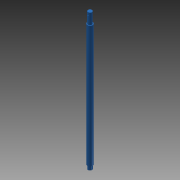
# Autodesk Inventor part: 砂轮轴
Saved by Autodesk Inventor 2015 (Build 190159000, 159)
## iProperties
Created: 2017-05-16
Part Number: 砂轮轴
Material: 常规
Document SubType Name: Modeling
Designer: Administrator
Density: 1 g/cm^3
Appearance: 青色
Author: Administrator
Autodesk Inventor part; units mm, degrees
ref_plane "YZ Plane" through (0, 0, 0) normal (1, 0, 0) x (0, 1, 0)
sketch "草图1" plane through (0, 0, 0) normal (0, 0, 1) x (1, 0, 0)
  circle A0 centre (0, 0) radius 10
  dimension "d0" = 20
  constraints: 1 centre point, 1 coincident
  measures "d0" diameter of A0
extrude "拉伸1" add sketch "草图1" along normal blind 450
sketch "草图2" plane through (0, 0, 450) normal (0, 0, 1) x (1, 0, 0)
  circle A0 centre (0, 0) radius 7.5
  dimension "d3" = 15
  constraints: 1 centre point, 1 coincident
  measures "d3" diameter of A0
extrude "拉伸2" add sketch "草图2" along normal blind 40
sketch "草图3" plane through (0, 0, 0) normal (0, 0, -1) x (-1, 0, 0)
  circle A0 centre (0, 0) radius 7.5
  dimension "d6" = 15
  constraints: 1 centre point, 1 coincident
  measures "d6" diameter of A0
extrude "拉伸3" add sketch "草图3" along normal blind 15
chamfer "倒角1" distance 0.5 angle 45 1 edges at (7.5, 0, -15)
ref_plane "工作平面1" through (0, 10, 0) normal (0, 1, 0) x (-1, 0, 0)
sketch "草图4" plane through (0, 10, 0) normal (0, 1, 0) x (-1, 0, 0)
  line L0 (3, 392) -> (-3, 392)
  line L1 (-3, 392) -> (-3, 408)
  line L2 (-3, 408) -> (3, 408)
  line L3 (3, 408) -> (3, 392)
  arc A0 (-3, 392) -> (3, 392) centre (0, 392) ccw
  arc A1 (3, 408) -> (-3, 408) centre (0, 408) ccw
  line L4 (10, 450) -> (-10, 450) projected
  point P0 (0, 0)
  dimension "d12" = 6
  dimension "d13" = 16
  dimension "d14" = 0
  dimension "d15" = 42
  constraints: 8 end point, 4 point on circle, 4 tangent, 2 centre point, 2 parallel, 1 horizontal, 1 perpendicular
  measures "d12" distance between parallel lines of L1 L3
  measures "d13" distance of L0.end L1.end
  measures "d14" horizontal distance of point (0, 0) A0.centre
  measures "d15" distance between parallel lines of L4 L2
extrude "拉伸4" cut sketch "草图4" against normal blind 2.5
pattern_linear "矩形阵列1" count 4 spacing 120 along (0, 0, -1) of "拉伸4"
ref_plane "工作平面2" through (0, -7.5, 450) normal (0, 1, 0) x (-1, 0, 0)
sketch "草图5" plane through (0, -7.5, 450) normal (0, 1, 0) x (-1, 0, 0)
  circle A0 centre (0, 30) radius 2
  line L0 (7.5, 40) -> (-7.5, 40) projected
  line L1 (0, -450) -> (0, -436.617)
  dimension "d21" = 4
  dimension "d22" = 10
  dimension "d23" = 13.383
  constraints: 2 end point, 1 centre point, 1 point on line, 1 vertical
  measures "d21" diameter of A0
  measures "d22" distance from line of L0 A0.centre
  measures "d23" distance of L1.start L1.end
extrude "拉伸5" cut sketch "草图5" along normal blind 1.5
